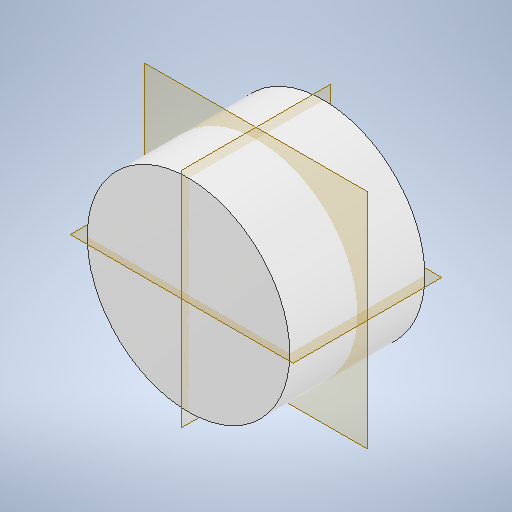
# Autodesk Inventor part: cilindro_0001_001
Saved by Autodesk Inventor 2025.2 (Build 292293000, 293)
## iProperties
Created: 2025-03-26
Part Number: cilindro_0001_001
Material: PCL plástico
Document SubType Name: Modeling
Designer: lucas
Density: 1.626 g/cm^3
Appearance: Suave - Branco
Author: lucas
Autodesk Inventor part; units mm, degrees
sketch "Esboço1" plane through (0, 0, 0) normal (0, 0, 1) x (1, 0, 0)
  circle A0 centre (0, 0) radius 7.5
  dimension "d0" = 15
  constraints: 1 centre point, 1 coincident
  measures "d0" diameter of A0
extrude "Extrusão1" add sketch "Esboço1" along normal mid plane 10
